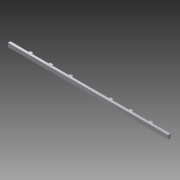
# Autodesk Inventor part: YRail
Saved by Autodesk Inventor 2015 (Build 190159000, 159)
## iProperties
Created: 2016-12-01
Part Number: YRail
Material: Generic
Document SubType Name: Modeling
Designer: Ernest
Density: 1 g/cm^3
Appearance: Default
Author: Ernest
Autodesk Inventor part; units mm, degrees
ref_plane "YZ Plane" through (0, 0, 0) normal (1, 0, 0) x (0, 1, 0)
ref_plane "XZ Plane" through (0, 0, 0) normal (0, 1, 0) x (-1, 0, 0)
ref_plane "XY Plane" through (0, 0, 0) normal (0, 0, 1) x (1, 0, 0)
sketch "Sketch1" plane through (0, 0, 0) normal (0, 0, 1) x (1, 0, 0)
  line L0 (0, 0) -> (2051, 0)
  line L1 (2051, 0) -> (2051, -30)
  line L2 (2051, -30) -> (0, -30)
  line L3 (0, -30) -> (0, 0)
  line L4 (256, 44.3402) -> (256, -8.0121) construction
  line L5 (512, 44.3402) -> (512, -8.0121) construction
  line L6 (768, 44.3402) -> (768, -8.0121) construction
  line L7 (1795, 15.5437) -> (1795, -11.3939) construction
  line L8 (1539, 15.5437) -> (1539, -11.3939) construction
  line L9 (1283, 15.5437) -> (1283, -11.3939) construction
  line L10 (236, 18.3) -> (276, 18.3)
  line L11 (276, 18.3) -> (276, 0)
  line L12 (276, 0) -> (236, 0)
  line L13 (236, 0) -> (236, 18.3)
  line L14 (492, 18.3) -> (532, 18.3)
  line L15 (532, 18.3) -> (532, 0)
  line L16 (532, 0) -> (492, 0)
  line L17 (492, 0) -> (492, 18.3)
  line L18 (748, 18.3) -> (788, 18.3)
  line L19 (788, 18.3) -> (788, 0)
  line L20 (788, 0) -> (748, 0)
  line L21 (748, 0) -> (748, 18.3)
  line L22 (1775, 18.3) -> (1815, 18.3)
  line L23 (1815, 18.3) -> (1815, 0)
  line L24 (1815, 0) -> (1775, 0)
  line L25 (1775, 0) -> (1775, 18.3)
  line L26 (1519, 18.3) -> (1559, 18.3)
  line L27 (1559, 18.3) -> (1559, 0)
  line L28 (1559, 0) -> (1519, 0)
  line L29 (1519, 0) -> (1519, 18.3)
  line L30 (1263, 18.3) -> (1303, 18.3)
  line L31 (1303, 18.3) -> (1303, 0)
  line L32 (1303, 0) -> (1263, 0)
  line L33 (1263, 0) -> (1263, 18.3)
  dimension "d0" = 2051
  dimension "d1" = 30
  dimension "d2" = 256
  dimension "d5" = 256
  dimension "d10" = 256
  dimension "d13" = 256
  dimension "d18" = 18.3
  dimension "d19" = 40
  dimension "d20" = 20
  dimension "d23" = 256
  dimension "d28" = 18.3
  dimension "d29" = 40
  dimension "d30" = 20
  dimension "d33" = 256
  constraints: 68 end point, 7 horizontal, 6 parallel, 4 perpendicular, 2 point on line, 1 vertical, 46 other
  measures "d0" distance of L1.end L2.end
  measures "d1" distance of L0.end L1.end
  measures "d2" distance between parallel lines of L3 L4
  measures "d5" distance of L4.start L5.start
  measures "d10" distance between parallel lines of L1 L7
  measures "d13" distance of L7.start L8.start
  measures "d18" distance between parallel lines of L0 L10
  measures "d19" distance between parallel lines of L11 L13
  measures "d20" distance between parallel lines of L11 L4
  measures "d23" distance of L11.end L15.end
  measures "d28" distance of L22.end L23.end
  measures "d29" distance of L22.start L22.end
  measures "d30" distance between parallel lines of L25 L7
  measures "d33" distance of L7.start point (1539, 15.544)
extrude "Extrusion1" add sketch "Sketch1" along normal blind 50
body "Solid1"
